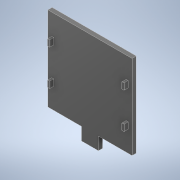
# Autodesk Inventor part: caixaled_pt2
Saved by Autodesk Inventor 2022 (Build 260153000, 153)
## iProperties
Created: 2024-02-25
Part Number: caixaled_pt2
Material: Plástico PC/ABS
Document SubType Name: Modeling
Designer: Daniel
Density: 0.357273 g/cm^3
Appearance: Suave - Preto
Author: Daniel
Autodesk Inventor part; units mm, degrees
ref_plane "YZ Plane" through (0, 0, 0) normal (1, 0, 0) x (0, 1, 0)
ref_plane "XZ Plane" through (0, 0, 0) normal (0, 1, 0) x (-1, 0, 0)
ref_plane "XY Plane" through (0, 0, 0) normal (0, 0, 1) x (1, 0, 0)
sketch "Esboço1" plane through (0, 0, 0) normal (0, 0, 1) x (1, 0, 0)
  line L0 (0, 0) -> (20, 0)
  line L1 (20, 0) -> (20, 20)
  line L2 (20, 20) -> (0, 20)
  line L3 (0, 20) -> (0, 0)
  dimension "d0" = 20
  dimension "d1" = 20
  constraints: 8 end point, 2 parallel, 1 horizontal, 1 perpendicular
  measures "d0" distance of L2.end L1.end
  measures "d1" distance of L1.end L0.end
extrude "Extrusão1" add sketch "Esboço1" along normal blind 1
sketch "Esboço2" plane through (0, 0, 1) normal (0, 0, 1) x (1, 0, 0)
  line L0 (0.9, 15) -> (1.4, 15)
  line L1 (1.4, 15) -> (1.4, 13.5)
  line L2 (1.4, 13.5) -> (0.9, 13.5)
  line L3 (0.9, 13.5) -> (0.9, 15)
  line L4 (0.9, 5) -> (1.4, 5)
  line L5 (1.4, 5) -> (1.4, 6.5)
  line L6 (1.4, 6.5) -> (0.9, 6.5)
  line L7 (0.9, 6.5) -> (0.9, 5)
  line L8 (0, 20) -> (0, 0) projected
  line L9 (0, 0) -> (20, 0) projected
  line L10 (20, 20) -> (0, 20) projected
  line L11 (10, 20) -> (10, 0)
  line L12 (19.1, 15) -> (18.6, 15)
  line L13 (18.6, 15) -> (18.6, 13.5)
  line L14 (18.6, 13.5) -> (19.1, 13.5)
  line L15 (19.1, 13.5) -> (19.1, 15)
  line L16 (19.1, 5) -> (18.6, 5)
  line L17 (18.6, 5) -> (18.6, 6.5)
  line L18 (18.6, 6.5) -> (19.1, 6.5)
  line L19 (19.1, 6.5) -> (19.1, 5)
  dimension "d4" = 1.5
  dimension "d5" = 0.5
  dimension "d6" = 0.5
  dimension "d7" = 1.5
  dimension "d8" = 0.9
  dimension "d9" = 5
  dimension "d10" = 5
  constraints: 34 end point, 8 symmetric about line, 4 parallel, 2 horizontal, 2 midpoint, 2 perpendicular, 2 point on line
  measures "d4" distance of L2.end L0.start
  measures "d5" distance of L0.start L0.end
  measures "d6" distance of L5.end L6.end
  measures "d7" distance of L6.end L4.start
  measures "d8" distance between parallel lines of L8 L3
  measures "d9" distance between parallel lines of L9 L4
  measures "d10" distance between parallel lines of L10 L0
extrude "Extrusão2" add sketch "Esboço2" along normal blind 1 contours L0 L1 L2 L3 | L7 L6 L5 L4 | L15 L14 L13 L12 | L16 L17 L18 L19
sketch "Esboço3" plane through (0, 0, 1) normal (0, 0, 1) x (1, 0, 0)
  line L0 (0, 0) -> (20, 0) projected
  line L1 (8, 0) -> (12, 0)
  line L2 (12, 0) -> (12, -3)
  line L3 (12, -3) -> (8, -3)
  line L4 (8, -3) -> (8, 0)
  dimension "d13" = 8
  dimension "d14" = 8
  dimension "d15" = 3
  constraints: 8 end point, 2 parallel, 1 horizontal, 1 perpendicular, 1 point on line
  measures "d13" distance from line of L0.start L4
  measures "d14" distance from line of L0.end L2
  measures "d15" distance of L1.end L2.end
extrude "Extrusão3" add sketch "Esboço3" against normal blind 1
